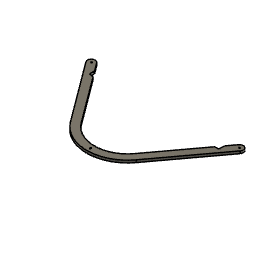
move_base_bumper_back (Autodesk Fusion 360 design; units mm, degrees)
Autodesk Fusion 360 part; units mm, degrees
note: some values were not read from the file. Set by a fixed rule: which sketch regions a step uses; the direction of a hole.
sketch "スケッチ1" plane through (0, 0, 0) normal (0, 1, 0) x (1, 0, 0)
  circle A0 centre (0, 0) radius 210
  circle A1 centre (0, -210) radius 85
  line L0 (68.3017, -260.5952) -> (168.7454, -125)
  line L1 (-168.7454, -125) -> (-68.3017, -260.5952)
  circle A2 centre (0, -210) radius 77
  circle A3 centre (0, -210) radius 69
  line L2 (61.8733, -255.8333) -> (154.1352, -131.2832)
  line L3 (55.4449, -251.0714) -> (147.7068, -126.5213)
  line L4 (-61.8733, -255.8333) -> (-154.1352, -131.2832)
  line L5 (-147.7068, -126.5213) -> (-55.4449, -251.0714)
  circle A4 centre (154.1352, -131.2832) radius 8
  circle A5 centre (-154.1352, -131.2832) radius 8
  line L6 (0, -210) -> (0, -295)
  line L7 (-135, 0) -> (135, 0)
  line L8 (135, 0) -> (135, -155)
  line L9 (135, -155) -> (-135, -155)
  line L10 (-135, -155) -> (-135, 0)
  point P0 (0, -287)
  dimension "d1" = 420
  dimension "d2" = 170
  dimension "d3" = 210
  dimension "d4" = 155
  dimension "d5" = 16
  dimension "d13" = 270
  dimension "d14" = 155
  constraint coincident A0.centre origin
  constraint vertical A0.centre A1.centre
  constraint tangent A0 L1
  constraint tangent A1 L1
  constraint tangent A1 L0
  constraint tangent A0 L0
  constraint coincident A0 L0.end
  constraint coincident A1 L0.start
  constraint coincident A1 L1.end
  constraint coincident A0 L1.start
  constraint concentric A1 A2
  constraint concentric A2 A3
  constraint parallel L2 L3
  constraint parallel L1 L4
  constraint tangent A2 L2
  constraint tangent A3 L3
  constraint tangent A3 L5
  constraint tangent A2 L4
  constraint coincident A2 L4.start
  constraint coincident A3 L5.end
  constraint coincident A3 L3.start
  constraint coincident A2 L2.start
  constraint parallel L0 L2
  constraint parallel L4 L5
  constraint coincident L2.end A4.centre
  constraint tangent L0 A4
  constraint coincident L4.end A5.centre
  constraint equal A4 A5
  constraint coincident L5.start A5
  constraint tangent L5 A5
  constraint coincident L3.end A4
  constraint equal L2 L4
  constraint coincident A1.centre A2.centre
  constraint coincident A1 L6.end
  constraint vertical L6
  constraint coincident L6 P0
  constraint coincident A2 P0
  constraint horizontal L7
  constraint vertical L8
  constraint horizontal L9
  constraint vertical L10
  constraint midpoint L7 A0.centre
  measures "d1" diameter of A0
  measures "d2" diameter of A1
  measures "d3" distance of A0.centre A1.centre
  measures "d4" distance of L2.start L2.end
  measures "d5" diameter of A4
  measures "d13" distance of L7.start L7.end
  measures "d14" distance of L7.start L9.end
extrude "押し出し1" add sketch "スケッチ1" along normal blind 5 contours A0 A5 | A0 A5 | A0 A1 L1 L4 A5 | A0 A4 | A0 A4 | A0 A1 L0 L2 A4 | A0 L4 A5 | A0 L4 L5 A5 L9 L10 | A1 A2 L4 L6 | A0 L2 A4 | A1 A2 L2 L6 | A0 A1 L4 L5 | A1 A2 L4 L5 | A0 A1 L2 L3 | A0 L2 L3 A4 L8 L9 | A1 A2 L2 L3 | A2 A3 L3 L6 | A2 A3 L5 L6
hole "穴1" at (0, 0, 287) at (-154.1352, 0, 131.2832) at (154.1352, 0, 131.2832) direction (0, 1, 0) diameter 3.2 end through all
fillet "フィレット1" radius 2 6 edges at (135, 2.5, 155) (-135, 2.5, 155) (126.6109, 2.5, 155) (135, 2.5, 143.675) (-135, 2.5, 143.675) (-126.6109, 2.5, 155)
